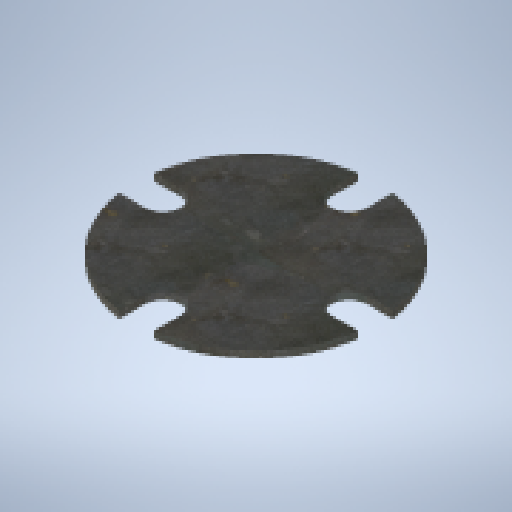
# Autodesk Inventor part: Base
Saved by Autodesk Inventor 2025.2 (Build 292293000, 293)
## iProperties
Created: 2025-04-01
Part Number: Base
Material: Steel
Document SubType Name: Modeling
Designer: bless
Density: 7.85 g/cm^3
Appearance: Plate
Author: bless
Autodesk Inventor part; units mm, degrees
ref_plane "YZ Plane" through (0, 0, 0) normal (1, 0, 0) x (0, 1, 0)
ref_plane "XZ Plane" through (0, 0, 0) normal (0, 1, 0) x (-1, 0, 0)
ref_plane "XY Plane" through (0, 0, 0) normal (0, 0, 1) x (1, 0, 0)
sketch "Sketch1" plane through (0, 0, 0) normal (0, 1, 0) x (-1, 0, 0)
  circle A0 centre (0, 0) radius 175
  dimension "d0" = 350
  constraints: 1 centre point, 1 coincident
  measures "d0" diameter of A0
extrude "Extrusion1" add sketch "Sketch1" along normal blind 10
sketch "Sketch2" plane through (0, 0, 0) normal (0, -1, 0) x (1, 0, 0)
  circle A0 centre (0, 0) radius 175 projected
  circle A1 centre (0, 135) radius 25
  line L0 (-25, 135) -> (-25, 173.2051)
  line L1 (25, 135) -> (25, 173.2051)
  dimension "d3" = 50
  dimension "d4" = 135
  constraints: 4 end point, 4 point on circle, 2 tangent, 1 centre point, 1 parallel, 1 vertical, 1 vertical alignment
  measures "d3" diameter of A1
  measures "d4" distance of A0.centre A1.centre
extrude "Extrusion2" cut sketch "Sketch2" against normal through all contours L1 A1 L0 A0 | A1 picked at (-14.0746, 168.7936)
pattern_circular "Circular Pattern1" count 4 over 360 about axis through (0, 0, 0) along (0, 1, 0) of "Extrusion2"
body "Solid1"
